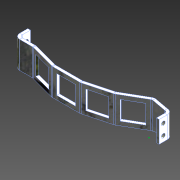
# Autodesk Inventor part: keyplate4
Saved by Autodesk Inventor 2018 (Build 220112000, 112)
## iProperties
Created: 2018-05-25
Part Number: keyplate4
Material: アルミニウム 6061
Document SubType Name: Sheet Metal
Designer: NaMACHAN
Density: 2.7 g/cm^3
Sheet Metal Rule: Al2mm
Appearance: アルミニウム - フラット
Mass: 8.56547 g
Surface Area: 42.6052 cm^2
Volume: 3.1724 cm^3
Author: NaMACHAN
Autodesk Inventor part; units mm, degrees
ref_plane "YZ Plane" through (0, 0, 0) normal (1, 0, 0) x (0, 1, 0)
ref_plane "XZ Plane" through (0, 0, 0) normal (0, 1, 0) x (-1, 0, 0)
ref_plane "XY Plane" through (0, 0, 0) normal (0, 0, 1) x (1, 0, 0)
sketch "スケッチ1" plane through (0, 0, 0) normal (0, 1, 0) x (-1, 0, 0)
  line L0 (-10, -10) -> (10, -10)
  line L1 (10, -10) -> (10, 10)
  line L2 (10, 10) -> (-10, 10)
  line L3 (-10, 10) -> (-10, -10)
  line L4 (-10, -10) -> (10, 10) construction
  line L5 (10, -10) -> (-10, 10) construction
  line L6 (-7, -7) -> (7, -7)
  line L7 (7, -7) -> (7, 7)
  line L8 (7, 7) -> (-7, 7)
  line L9 (-7, 7) -> (-7, -7)
  line L10 (-7, -7) -> (7, 7) construction
  line L11 (7, -7) -> (-7, 7) construction
  point P0 (0, 0)
  dimension "d0" = 20
  dimension "d1" = 20
  dimension "d2" = 14
  dimension "d3" = 14
  measures "d0" distance of L2.end L1.end
  measures "d1" distance of L1.end L0.end
  measures "d2" distance of L8.end L7.end
  measures "d3" distance of L7.end L6.end
extrude "プレート1" add sketch "スケッチ1" along normal blind 2
sketch "スケッチ2" plane through (-10.5176, 2.0681, 10) normal (-0.258819, -0.9659258, 0) x (0.9659258, -0.258819, 0)
  line L0 (0, -20) -> (0, 0)
  line L1 (0, 0) -> (-19.4734, 0)
  line L2 (-19.4734, 0) -> (-19.4734, -20)
  line L3 (-19.4734, -20) -> (0, -20)
  constraints: 6 end point, 1 horizontal, 1 perpendicular, 1 vertical
edge flange "フランジ1" height 20 angle 15 thickness 2 bend radius 2 thickness toward (-0.258819, -0.9659258, 0) relief straight relief width 2 relief depth 1 edges at (-10, 2, 0) wall of the first edge with corners at (-10.5176, 2.0681, -10) (-10.5176, 2.0681, 10) (-29.3275, 7.1082, 10) (-29.3275, 7.1082, -10)
bend "曲げ1"
corner "コーナー1"
sketch "スケッチ3" plane through (10.5176, 2.0681, -10) normal (0.258819, -0.9659258, 0) x (0.9659258, 0.258819, 0)
  line L0 (0, 20) -> (0, 0)
  line L1 (0, 0) -> (19.4734, 0)
  line L2 (19.4734, 0) -> (19.4734, 20)
  line L3 (19.4734, 20) -> (0, 20)
  constraints: 6 end point, 1 horizontal, 1 perpendicular, 1 vertical
edge flange "フランジ2" height 20 angle 15 thickness 2 bend radius 2 thickness toward (0.258819, -0.9659258, 0) relief straight relief width 2 relief depth 1 edges at (10, 2, 0) wall of the first edge with corners at (10.5176, 2.0681, 10) (10.5176, 2.0681, -10) (29.3275, 7.1082, -10) (29.3275, 7.1082, 10)
bend "曲げ2"
corner "コーナー2"
sketch "スケッチ4" plane through (29.8099, 7.308, -10) normal (0.5, -0.8660254, 0) x (0.8660254, 0.5, 0)
  line L0 (0, 20) -> (0, 0)
  line L1 (0, 0) -> (19.4734, 0)
  line L2 (19.4734, 0) -> (19.4734, 20)
  line L3 (19.4734, 20) -> (0, 20)
  constraints: 6 end point, 1 horizontal, 1 perpendicular, 1 vertical
edge flange "フランジ3" height 20 angle 15 thickness 2 bend radius 2 thickness toward (0.5, -0.8660254, 0) relief straight relief width 2 relief depth 1 edges at (29.3275, 7.1082, 0) wall of the first edge with corners at (29.8099, 7.308, 10) (29.8099, 7.308, -10) (46.6743, 17.0447, -10) (46.6743, 17.0447, 10)
bend "曲げ3"
corner "コーナー3"
sketch "スケッチ5" plane through (48.6743, 15.5806, -10) normal (0, 1, 0) x (1, 0, 0)
  line L0 (0, 20) -> (0, 0)
  line L1 (0, 0) -> (8.9282, 0)
  line L2 (8.9282, 0) -> (8.9282, 20)
  line L3 (8.9282, 20) -> (0, 20)
  constraints: 6 end point, 1 horizontal, 1 perpendicular, 1 vertical
edge flange "フランジ4" height 10 angle -30 thickness 2 bend radius 2 thickness toward (0, 1, 0) relief straight relief width 2 relief depth 1 edges at (46.6743, 17.0447, 0) wall of the first edge with corners at (48.6743, 15.5806, 10) (48.6743, 15.5806, -10) (57.6025, 15.5806, -10) (57.6025, 15.5806, 10)
bend "曲げ4"
corner "コーナー4"
sketch "スケッチ6" plane through (-30.3628, 5.2445, 10) normal (0, 1, 0) x (1, 0, 0)
  line L0 (0, -20) -> (0, 0)
  line L1 (0, 0) -> (-9.4734, 0)
  line L2 (-9.4734, 0) -> (-9.4734, -20)
  line L3 (-9.4734, -20) -> (0, -20)
  constraints: 6 end point, 1 horizontal, 1 perpendicular, 1 vertical
edge flange "フランジ5" height 10 angle -15 thickness 2 bend radius 2 thickness toward (0, 1, 0) relief straight relief width 2 relief depth 1 edges at (-29.3275, 7.1082, 0) wall of the first edge with corners at (-30.3628, 5.2445, -10) (-30.3628, 5.2445, 10) (-39.8362, 5.2445, 10) (-39.8362, 5.2445, -10)
bend "曲げ5"
corner "コーナー5"
sketch "スケッチ7" plane through (10.5176, 2.0681, 10) normal (-0.258819, 0.9659258, 0) x (0.9659258, 0.258819, 0)
  line L0 (2.7367, 17) -> (16.7367, 17)
  line L1 (16.7367, 17) -> (16.7367, 3)
  line L2 (16.7367, 3) -> (2.7367, 3)
  line L3 (2.7367, 3) -> (2.7367, 17)
  line L4 (2.7367, 17) -> (16.7367, 3) construction
  line L5 (16.7367, 17) -> (2.7367, 3) construction
  line L6 (19.4734, 0) -> (0, 0) projected
  line L7 (-0.5176, 20) -> (-0.5176, 0) projected
  point P0 (-10.6945, 10)
  point P1 (9.7367, 10)
  point P2 (9.7367, 10)
  point P3 (9.7367, 0)
  point P4 (9.7367, 10)
  point P5 (-0.5176, 10)
  dimension "d55" = 14
  dimension "d56" = 14
  constraints: 12 end point, 6 midpoint, 2 parallel, 1 horizontal, 1 horizontal alignment, 1 perpendicular, 1 vertical alignment
  measures "d55" distance of L1.end L2.end
  measures "d56" distance of L0.end L1.end
extrude "押し出し1" cut sketch "スケッチ7" against normal blind 10
sketch "スケッチ8" plane through (29.8099, 7.308, 10) normal (-0.5, 0.8660254, 0) x (0.8660254, 0.5, 0)
  line L0 (2.7367, 17) -> (16.7367, 17)
  line L1 (16.7367, 17) -> (16.7367, 3)
  line L2 (16.7367, 3) -> (2.7367, 3)
  line L3 (2.7367, 3) -> (2.7367, 17)
  line L4 (2.7367, 17) -> (16.7367, 3) construction
  line L5 (16.7367, 17) -> (2.7367, 3) construction
  line L6 (-0.5176, 0) -> (-0.5176, 20) projected
  line L7 (19.4734, 0) -> (0, 0) projected
  point P0 (-29.4701, 10)
  point P1 (9.7367, 10)
  point P2 (9.7367, 10)
  point P3 (-0.5176, 10)
  point P4 (9.7367, 10)
  point P5 (9.7367, 0)
  dimension "d59" = 14
  dimension "d60" = 14
  constraints: 12 end point, 6 midpoint, 2 parallel, 1 horizontal, 1 horizontal alignment, 1 perpendicular, 1 vertical alignment
  measures "d59" distance of L1.end L2.end
  measures "d60" distance of L0.end L1.end
extrude "押し出し2" cut sketch "スケッチ8" against normal blind 10
sketch "スケッチ9" plane through (-10.5176, 2.0681, 10) normal (0.258819, 0.9659258, 0) x (0.9659258, -0.258819, 0)
  line L0 (-16.7367, 17) -> (-2.7367, 17)
  line L1 (-2.7367, 17) -> (-2.7367, 3)
  line L2 (-2.7367, 3) -> (-16.7367, 3)
  line L3 (-16.7367, 3) -> (-16.7367, 17)
  line L4 (-16.7367, 17) -> (-2.7367, 3) construction
  line L5 (-2.7367, 17) -> (-16.7367, 3) construction
  line L6 (-19.4734, 20) -> (-19.4734, 0) projected
  line L7 (-19.4734, 0) -> (0, 0) projected
  point P0 (10.6945, 10)
  point P1 (-9.7367, 10)
  point P2 (-9.7367, 10)
  point P3 (-19.4734, 10)
  point P4 (-9.7367, 10)
  point P5 (-9.7367, 0)
  dimension "d63" = 14
  dimension "d64" = 14
  constraints: 12 end point, 6 midpoint, 2 parallel, 1 horizontal, 1 horizontal alignment, 1 perpendicular, 1 vertical alignment
  measures "d63" distance of L1.end L2.end
  measures "d64" distance of L0.end L1.end
extrude "押し出し3" cut sketch "スケッチ9" against normal blind 10
sketch "スケッチ19" plane through (57.6025, 17.5806, 10) normal (0, 1, 0) x (1, 0, 0)
  line L0 (0, 0) -> (0, 20) projected
  line L1 (0, 20) -> (0, 18)
  line L2 (-8.9282, 20) -> (-8.9282, 0) projected
  line L3 (-8.9282, 20) -> (0, 20)
  line L4 (0, 20) -> (-8.9282, 20) projected
  line L5 (0, 18) -> (-8.9282, 20)
  line L6 (0, 0) -> (0, 2)
  line L7 (-8.9282, 0) -> (-10.9282, 0) projected
  line L8 (-8.9282, 0) -> (0, 2)
  line L9 (0, 0) -> (-8.9282, 0)
  point P0 (-57.6025, 10)
  dimension "d140" = 2
  dimension "d141" = 2
  constraints: 12 end point, 2 perpendicular, 2 point on line
  measures "d140" distance of L0.end L1.end
  measures "d141" distance of L0.start L6.end
extrude "押し出し9" cut sketch "スケッチ19" against normal blind 10 contours L9 L8 L0 | L5 L3 L0
sketch "スケッチ20" plane through (59.6025, 13.5806, 8) normal (1, 0, 0) x (0, 1, 0)
  line L0 (0, -16) -> (0, 0)
  line L1 (0, 0) -> (-6, 0)
  line L2 (-6, 0) -> (-6, -16)
  line L3 (-6, -16) -> (0, -16)
  constraints: 6 end point, 1 horizontal, 1 perpendicular, 1 vertical
edge flange "フランジ10" height 10 angle 90 thickness 2 bend radius 2 thickness toward (1, 0, 0) relief straight relief width 2 relief depth 1 edges at (57.6025, 15.5806, 0) wall of the first edge with corners at (59.6025, 13.5806, -8) (59.6025, 13.5806, 8) (59.6025, 7.5806, 8) (59.6025, 7.5806, -8)
bend "曲げ10"
corner "コーナー10"
sketch "スケッチ21" plane through (-41.8362, 9.2445, -10) normal (-1, 0, 0) x (0, 1, 0)
  line L0 (0, 20) -> (0, 0)
  line L1 (0, 0) -> (6, 0)
  line L2 (6, 0) -> (6, 20)
  line L3 (6, 20) -> (0, 20)
  constraints: 8 end point
edge flange "フランジ11" height 10 angle -90 thickness 2 bend radius 2 thickness toward (-1, 0, 0) relief straight relief width 2 relief depth 1 edges at (-39.8362, 5.2445, 0) wall of the first edge with corners at (-41.8362, 9.2445, 10) (-41.8362, 9.2445, -10) (-41.8362, 15.2445, -10) (-41.8362, 15.2445, 10)
bend "曲げ11"
corner "コーナー11"
sketch "スケッチ22" plane through (61.6025, 7.5806, 8) normal (1, 0, 0) x (0, 0, -1)
  point P0 (8, -7.5806)
sketch "スケッチ24" plane through (61.6025, 7.5806, 8) normal (1, 0, 0) x (0, 0, -1)
  line L0 (16, 6) -> (16, 0) projected
  line L1 (0, 0) -> (0, 6) projected
  point P0 (8, -7.5806)
  point P1 (4, 3)
  point P2 (12, 3)
  point P3 (0, 3)
  dimension "d173" = 4
  dimension "d174" = 4
  constraints: 2 horizontal alignment, 1 midpoint
  measures "d173" distance from line of L0 point (12, 3)
  measures "d174" distance from line of L1 point (4, 3)
hole "穴2" at (61.6025, 10.5806, -4) at (61.6025, 10.5806, 4) direction (-1, 0, 0) diameter 3 depth 2 tip angle 118
sketch "スケッチ25" plane through (-41.8362, 15.2445, -10) normal (1, 0, 0) x (0, 0, 1)
  line L0 (20, 6) -> (20, 0) projected
  line L1 (0, 0) -> (0, 6) projected
  point P0 (10, 15.2445)
  point P1 (6, 3)
  point P2 (14, 3)
  point P3 (0, 3)
  dimension "d182" = 6
  dimension "d183" = 6
  constraints: 2 horizontal alignment, 1 midpoint
  measures "d182" distance from line of L0 point (14, 3)
  measures "d183" distance from line of L1 point (6, 3)
hole "穴3" at (-41.8362, 12.2445, -4) at (-41.8362, 12.2445, 4) direction (-1, 0, 0) diameter 3 depth 2 tip angle 118
equation "\"d180\" = Thickness"
equation "\"d189\" = Thickness"
equation "\"d4\" = Thickness"
equation "\"d5\" = BendReliefWidth"
equation "\"d6\" = BendReliefDepth"
equation "\"d7\" = MinimumRemnant"
equation "\"d8\" = TransitionRadius"
equation "\"d11\" = BendRadius"
equation "\"d12\" = CornerReliefSize"
equation "\"d13\" = GapSize"
equation "\"d14\" = JacobiRadiusSize"
equation "\"d15\" = BendReliefWidth"
equation "\"d16\" = BendReliefDepth"
equation "\"d17\" = MinimumRemnant"
equation "\"d18\" = TransitionRadius"
equation "\"d21\" = BendRadius"
equation "\"d22\" = CornerReliefSize"
equation "\"d23\" = GapSize"
equation "\"d24\" = JacobiRadiusSize"
equation "\"d25\" = BendReliefWidth"
equation "\"d26\" = BendReliefDepth"
equation "\"d27\" = MinimumRemnant"
equation "\"d28\" = TransitionRadius"
equation "\"d31\" = BendRadius"
equation "\"d32\" = CornerReliefSize"
equation "\"d33\" = GapSize"
equation "\"d34\" = JacobiRadiusSize"
equation "\"d35\" = BendReliefWidth"
equation "\"d36\" = BendReliefDepth"
equation "\"d37\" = MinimumRemnant"
equation "\"d38\" = TransitionRadius"
equation "\"d41\" = BendRadius"
equation "\"d42\" = CornerReliefSize"
equation "\"d43\" = GapSize"
equation "\"d44\" = JacobiRadiusSize"
equation "\"d45\" = BendReliefWidth"
equation "\"d46\" = BendReliefDepth"
equation "\"d47\" = MinimumRemnant"
equation "\"d48\" = TransitionRadius"
equation "\"d51\" = BendRadius"
equation "\"d52\" = CornerReliefSize"
equation "\"d53\" = GapSize"
equation "\"d54\" = JacobiRadiusSize"
equation "\"d144\" = BendReliefWidth"
equation "\"d145\" = BendReliefDepth"
equation "\"d146\" = MinimumRemnant"
equation "\"d147\" = TransitionRadius"
equation "\"d150\" = BendRadius"
equation "\"d151\" = CornerReliefSize"
equation "\"d152\" = GapSize"
equation "\"d153\" = JacobiRadiusSize"
equation "\"d154\" = BendReliefWidth"
equation "\"d155\" = BendReliefDepth"
equation "\"d156\" = MinimumRemnant"
equation "\"d157\" = TransitionRadius"
equation "\"d160\" = BendRadius"
equation "\"d161\" = CornerReliefSize"
equation "\"d162\" = GapSize"
equation "\"d163\" = JacobiRadiusSize"
equation "\"BendRadius\" = Thickness"
equation "\"BendReliefWidth\" = Thickness"
equation "\"BendReliefDepth\" = 0.5 * Thickness"
equation "\"CornerReliefSize\" = 4 * Thickness"
equation "\"MinimumRemnant\" = 2 * Thickness"
equation "\"TransitionRadius\" = BendRadius"
equation "\"JacobiRadiusSize\" = BendRadius"
equation "\"GapSize\" = Thickness"
equation "\"Thickness\" = 2"
